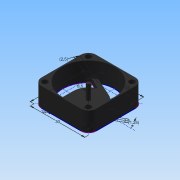
# Autodesk Inventor part: кулер корпус
Saved by Autodesk Inventor 2017 (Build 210142000, 142)
## iProperties
Part Number: кулер корпус
Material: Типовые
Document SubType Name: Modeling
Designer: alcapone
Density: 1 g/cm^3
Appearance: Резина — черная
Mass: 2.74841 g
Surface Area: 37.2355 cm^2
Volume: 2.74841 cm^3
Author: alcapone
Autodesk Inventor part; units mm, degrees
ref_plane "YZ Plane" through (0, 0, 0) normal (1, 0, 0) x (0, 1, 0)
ref_plane "XZ Plane" through (0, 0, 0) normal (0, 1, 0) x (-1, 0, 0)
ref_plane "XY Plane" through (0, 0, 0) normal (0, 0, 1) x (1, 0, 0)
sketch "Эскиз1" plane through (0, 0, 0) normal (0, 0, 1) x (1, 0, 0)
  line L0 (0, 0) -> (0, 15) construction
  line L1 (0, 0) -> (-22.981013, 0) construction
  line L2 (10.85, 15) -> (-10.85, 15)
  line L3 (-15, 10.85) -> (-15, -10.85)
  line L4 (-10.85, -15) -> (10.85, -15)
  line L5 (15, -10.85) -> (15, 10.85)
  line L6 (15, 15) -> (-15, -15) construction
  line L7 (-15, 15) -> (15, -15) construction
  circle A0 centre (0, 0) radius 14.4
  line L8 (-12, -12) -> (12, -12) construction
  line L9 (12, -12) -> (12, 12) construction
  line L10 (12, 12) -> (-12, 12) construction
  line L11 (-12, 12) -> (-12, -12) construction
  line L12 (-12, -12) -> (12, 12) construction
  line L13 (12, -12) -> (-12, 12) construction
  circle A1 centre (12, 12) radius 1.5
  circle A2 centre (-12, 12) radius 1.5
  circle A3 centre (-12, -12) radius 1.5
  circle A4 centre (12, -12) radius 1.5
  arc A5 (15, 10.85) -> (10.85, 15) centre (10.85, 10.85) ccw
  arc A6 (-10.85, 15) -> (-15, 10.85) centre (-10.85, 10.85) ccw
  arc A7 (-15, -10.85) -> (-10.85, -15) centre (-10.85, -10.85) ccw
  arc A8 (10.85, -15) -> (15, -10.85) centre (10.85, -10.85) ccw
  line L14 (0, 0) -> (26.197647, 0) construction
  line L15 (14.322508, -1.491896) -> (4.279514, -7.344097)
  line L16 (14.331135, 1.406612) -> (8.222871, -2.152764)
  line L17 (14.4, 0) -> (7.870044, -3.805102) construction
  line L18 (-7.13266, -13.861758) -> (-7.204633, -5.378159) construction
  line L19 (-8.370965, 11.716951) -> (-0.710884, 8.270069) construction
  line L20 (-8.401084, -11.695375) -> (-8.500306, 0)
  line L21 (-5.948706, -6.071482) -> (-5.888731, -13.140885)
  line L22 (3.48797, 7.751391) -> (-7.111996, 12.521162)
  line L23 (-3.02844, 7.942201) -> (-9.475461, 10.84323)
  arc A9 (8.222871, -2.152764) -> (3.48797, 7.751391) centre (0, 0) ccw
  arc A10 (-3.02844, 7.942201) -> (-8.5, 0) centre (0, 0) ccw
  arc A11 (-5.948706, -6.071482) -> (4.279514, -7.344097) centre (0, 0) ccw
  arc A12 (14.322508, -1.491896) -> (14.331135, 1.406612) centre (0, 0) ccw
  arc A13 (-8.401084, -11.695375) -> (-5.888731, -13.140885) centre (0, 0) ccw
  arc A14 (-7.111996, 12.521162) -> (-9.475461, 10.84323) centre (0, 0) ccw
  arc A15 (14.322508, -1.491896) -> (14.331135, 1.406612) centre (0, 0) ccw
  arc A16 (-9.475461, 10.84323) -> (-8.401084, -11.695375) centre (0, 0) ccw
  line L24 (-9.475461, 10.84323) -> (-3.02844, 7.942201)
  line L25 (-8.500306, 0) -> (-8.401084, -11.695375)
  line L26 (-5.948706, -6.071482) -> (-5.888731, -13.140885)
  arc A17 (-8.401084, -11.695375) -> (-5.888731, -13.140885) centre (0, 0) ccw
  arc A18 (-9.475461, 10.84323) -> (-5.888731, -13.140885) centre (0, 0) ccw
  arc A19 (-7.111996, 12.521162) -> (-8.401084, -11.695375) centre (0, 0) ccw
  point P0 (-0.367875, -0.714936)
  dimension "d24" = 360
  dimension "d52" = 28.8
  dimension "d0" = 30
  dimension "d1" = 30
  dimension "d8" = 3
  dimension "d9" = 3
  dimension "d10" = 3
  dimension "d11" = 3
  dimension "d19" = 2.5
  dimension "d26" = 1.25
  dimension "d27" = 2.5
  dimension "d28" = 1.25
  dimension "d32" = 2.5
  dimension "d33" = 1.25
  dimension "d49" = 8.5
  dimension "d50" = 8.5
  dimension "d51" = 8.5
  dimension "d53" = 24
  constraints: 54 end point, 31 point on circle, 19 centre point, 14 tangent, 12 point on line, 9 coincident, 9 parallel, 4 horizontal, 4 midpoint, 3 equal radius, 2 collinear, 2 perpendicular, 1 vertical, 22 other
  measures "d0" distance of L7.end L6.end
  measures "d1" distance of L6.end L7.start
  measures "d8" diameter of A1
  measures "d9" diameter of A2
  measures "d10" diameter of A3
  measures "d11" diameter of A4
  measures "d19" distance between parallel lines of L15 L16
  measures "d26" distance between parallel lines of L20 L18
  measures "d27" distance between parallel lines of L20 L21
  measures "d28" distance between parallel lines of L19 L22
  measures "d32" distance between parallel lines of L23 L22
  measures "d33" distance between parallel lines of L15 L17
  measures "d49" radius of A9
  measures "d50" radius of A10
  measures "d51" radius of A11
  measures "d53" distance of L9.end L10.end
extrude "Выдавливание2" add sketch "Эскиз1" along normal blind 10.5 contours A5 L5 A8 L4 A7 L3 A6 L2 | A1 | A2 | A3 | A4
extrude "Выдавливание3" add sketch "Эскиз1" along normal blind 2 contours A0 L15 A11 L21 L20 A10 L23 L22 A9 L16 | L23 A10 L20 A0
sketch "Эскиз2" plane through (0, 0, 2) normal (0, 0, 1) x (1, 0, 0)
  circle A0 centre (0, 0) radius 1
  dimension "d45" = 2
  constraints: 1 centre point, 1 coincident
  measures "d45" diameter of A0
extrude "Выдавливание6" add sketch "Эскиз2" along normal blind 8
sketch "Эскиз3" plane through (0, 0, 2) normal (0, 0, 1) x (1, 0, 0)
  line L0 (0.220979, -0.099936) -> (0.220979, 15) construction
  line L1 (0.220979, -0.099936) -> (-22.981013, -0.099936) construction
  line L2 (10.85, 14.900064) -> (-10.408041, 14.900064)
  line L3 (-14.779021, 10.529085) -> (-14.779021, -10.728956)
  line L4 (-10.408041, -15.099936) -> (10.85, -15.099936)
  line L5 (15.220979, -10.728956) -> (15.220979, 10.529085)
  line L6 (15.220979, 14.900064) -> (-14.779021, -15.099936) construction
  line L7 (-14.779021, 14.900064) -> (15.220979, -15.099936) construction
  line L8 (-11.779021, -12.099936) -> (12.220979, -12.099936) construction
  line L9 (12.220979, -12.099936) -> (12.220979, 11.900064) construction
  line L10 (12.220979, 11.900064) -> (-11.779021, 11.900064) construction
  line L11 (-11.779021, 11.900064) -> (-11.779021, -12.099936) construction
  line L12 (-11.779021, -12.099936) -> (12.220979, 11.900064) construction
  line L13 (12.220979, -12.099936) -> (-11.779021, 11.900064) construction
  circle A0 centre (12.220979, 11.900064) radius 1.75
  circle A1 centre (-11.779021, 11.900064) radius 1.75
  circle A2 centre (-11.779021, -12.099936) radius 1.75
  circle A3 centre (12.220979, -12.099936) radius 1.75
  arc A4 (15.220979, 10.529085) -> (10.85, 14.900064) centre (10.85, 10.529085) ccw
  arc A5 (-10.408041, 14.900064) -> (-14.779021, 10.529085) centre (-10.408041, 10.529085) ccw
  arc A6 (-14.779021, -10.728956) -> (-10.408041, -15.099936) centre (-10.408041, -10.728956) ccw
  arc A7 (10.85, -15.099936) -> (15.220979, -10.728956) centre (10.85, -10.728956) ccw
  line L14 (0.220979, -0.099936) -> (26.197647, -0.099936) construction
  line L15 (14.765082, -1.58245) -> (4.43625, -7.481094)
  line L16 (14.773156, 1.301112) -> (8.424753, -2.324366)
  line L17 (14.840445, -0.099936) -> (7.933925, -4.044147) construction
  line L18 (-7.029021, -14.080975) -> (-7.029021, -5.340351) construction
  line L19 (-8.202223, 11.849057) -> (-0.585826, 8.283092) construction
  line L20 (-8.279021, -11.994421) -> (-8.279021, -0.099936)
  line L21 (-5.779021, -6.120733) -> (-5.779021, -13.431431)
  line L22 (3.825169, 7.598104) -> (-6.947092, 12.641631)
  line L23 (-2.687632, 7.886927) -> (-9.308579, 10.986827)
  arc A8 (8.424753, -2.324366) -> (3.825169, 7.598104) centre (0.220979, -0.099936) ccw
  arc A9 (-2.687632, 7.886927) -> (-8.279021, -0.099936) centre (0.220979, -0.099936) ccw
  arc A10 (-5.779021, -6.120733) -> (4.43625, -7.481094) centre (0.220979, -0.099936) ccw
  arc A11 (14.765082, -1.58245) -> (14.773156, 1.301112) centre (0.441536, -0.100553) ccw
  arc A12 (-6.947092, 12.641631) -> (-8.202223, 11.849057) centre (0.103647, 0.085873) ccw
  arc A13 (14.765082, -1.58245) -> (14.773156, 1.301112) centre (0.441536, -0.100553) ccw
  line L24 (-9.308579, 10.986827) -> (-2.687632, 7.886927)
  line L25 (-8.279021, -0.099936) -> (-8.279021, -11.994421)
  line L26 (-5.779021, -6.120733) -> (-5.779021, -13.431431)
  arc A14 (-6.947092, 12.641631) -> (-8.202223, 11.849057) centre (0.220979, -0.099936) ccw
  arc A15 (-9.308579, 10.986827) -> (-8.279021, -11.994421) centre (0.220979, -0.099936) ccw
  arc A16 (-10.116544, -10.437459) -> (-7.029021, -12.795064) centre (0.220979, -0.099936) ccw
  arc A17 (-7.029021, -12.795064) -> (-5.779021, -13.431431) centre (0.220979, -0.099936) ccw
  arc A18 (-7.029021, -12.795064) -> (-8.202223, 11.849057) centre (0.220979, -0.099936) ccw
  arc A19 (-7.029021, -12.795064) -> (-5.779021, -13.431431) centre (0.121294, -0.295744) ccw
  arc A20 (-11.779021, -8.450312) -> (-5.779021, -13.431431) centre (0.220979, -0.099936) ccw
  arc A21 (-7.029021, -12.795064) -> (-5.779021, -13.431431) centre (0.220979, -0.099936) ccw
  circle A22 centre (0, 0) radius 14.4
  point P0 (-0.130266, -0.777285)
  dimension "d73" = 360
  dimension "d56" = 30
  dimension "d57" = 30
  dimension "d58" = 3.5
  dimension "d59" = 3.5
  dimension "d60" = 3.5
  dimension "d61" = 3.5
  dimension "d62" = 2.5
  dimension "d63" = 1.25
  dimension "d64" = 2.5
  dimension "d65" = 1.25
  dimension "d66" = 2.5
  dimension "d67" = 1.25
  dimension "d68" = 8.5
  dimension "d69" = 8.5
  dimension "d70" = 8.5
  dimension "d72" = 24
  dimension "d78" = 14.61947
  constraints: 54 end point, 47 point on circle, 22 centre point, 14 point on line, 11 tangent, 9 coincident, 9 parallel, 4 horizontal, 4 midpoint, 3 equal radius, 2 collinear, 2 perpendicular, 1 vertical, 11 other
  measures "d56" distance of L7.end L6.end
  measures "d57" distance of L6.end L7.start
  measures "d58" diameter of A0
  measures "d59" diameter of A1
  measures "d60" diameter of A2
  measures "d61" diameter of A3
  measures "d62" distance between parallel lines of L15 L16
  measures "d63" distance between parallel lines of L20 L18
  measures "d64" distance between parallel lines of L20 L21
  measures "d65" distance between parallel lines of L19 L22
  measures "d66" distance between parallel lines of L23 L22
  measures "d67" distance between parallel lines of L15 L17
  measures "d68" radius of A8
  measures "d69" radius of A9
  measures "d70" radius of A10
  measures "d72" distance of L9.end L10.end
  measures "d78" radius of A15
sketch "Эскиз3 outline for Выдавливание7" plane through (0, 0, 2) normal (0, 0, 1) x (1, 0, 0)
  line L0 (-8.279021, -11.994421) -> (-8.279021, -0.099936)
  arc A0 (-10.116544, -10.437459) -> (-8.279021, -11.994421) centre (0.220979, -0.099936) ccw
  arc A1 (-11.779021, -8.450312) -> (-10.116544, -10.437459) centre (0.220979, -0.099936) ccw
  arc A2 (-9.308579, 10.986827) -> (-11.779021, -8.450312) centre (0.220979, -0.099936) ccw
  line L1 (-2.687632, 7.886927) -> (-9.308579, 10.986827)
  arc A3 (-8.279021, -0.099936) -> (-2.687632, 7.886927) centre (0.220979, -0.099936) cw
extrude "Выдавливание7" cut sketch "Эскиз3 outline for Выдавливание7" against normal blind 10
extrude "Выдавливание8" cut sketch "Эскиз1" along normal blind 20 contours A1 | A2 | A3 | A4
